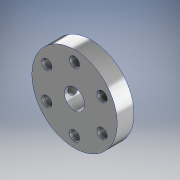
# Autodesk Inventor part: motor_axle_mounting_hub_6_mm
Saved by Autodesk Inventor 2016 (Build 200138000, 138)
## iProperties
Created: 2016-04-24
Part Number: motor_axle_mounting_hub_6_mm
Material: Aluminum 6061
Document SubType Name: Modeling
Designer: Henrik Samuelsson
Density: 2.7 g/cm^3
Appearance: Aluminum - Flat
Author: Henrik Samuelsson
Autodesk Inventor part; units mm, degrees
ref_plane "YZ Plane" through (0, 0, 0) normal (1, 0, 0) x (0, 1, 0)
ref_plane "XZ Plane" through (0, 0, 0) normal (0, 1, 0) x (-1, 0, 0)
ref_plane "XY Plane" through (0, 0, 0) normal (0, 0, 1) x (1, 0, 0)
sketch "Sketch1" plane through (0, 0, 0) normal (0, 1, 0) x (-1, 0, 0)
  circle A0 centre (0, 0) radius 12.7
  circle A1 centre (8.2272, -4.75) radius 1.5
  circle A2 centre (8.2272, 4.75) radius 1.5
  circle A3 centre (0, 9.5) radius 1.5
  circle A4 centre (-8.2272, 4.75) radius 1.5
  circle A5 centre (-8.2272, -4.75) radius 1.5
  circle A6 centre (0, -9.5) radius 1.5
  dimension "d0" = 25.4
  dimension "d1" = 3
  dimension "d3" = 9.5
  dimension "d6" = 360
  dimension "d20" = 0
  constraints: 7 centre point, 3 coincident, 17 other
  measures "d0" diameter of A0
  measures "d1" diameter of A1
  measures "d3" distance of A1.centre point (0, 0)
  measures "d20" horizontal distance of point (0, 0) A6.centre
extrude "Extrusion1" add sketch "Sketch1" along normal blind 5
sketch "Sketch2" plane through (0, 0, 0) normal (0, 1, 0) x (-1, 0, 0)
  circle A0 centre (0, 0) radius 3
  dimension "d10" = 6
  constraints: 1 centre point, 1 coincident
  measures "d10" diameter of A0
extrude "Extrusion2" cut sketch "Sketch2" along normal through all
sketch "Sketch3" plane through (0, 5, 0) normal (0, 1, 0) x (1, 0, 0)
  circle A0 centre (0, 0) radius 3
  circle A1 centre (0, 0) radius 6
  dimension "d13" = 12
  constraints: 2 centre point, 2 coincident
  measures "d13" diameter of A1
extrude "Extrusion3" add sketch "Sketch3" along normal blind 4.2
sketch "Sketch5" plane through (0, 0, 0) normal (1, 0, 0) x (0, 1, 0)
  circle A0 centre (2.5, 0) radius 1.5
  point P0 (0, 0)
  dimension "d21" = 3
  dimension "d22" = 2.5
  dimension "d23" = 0
  constraints: 1 centre point
  measures "d21" diameter of A0
  measures "d22" distance of point (0, 0) A0.centre
  measures "d23" vertical distance of point (0, 0) A0.centre
extrude "Extrusion4" cut sketch "Sketch5" against normal through all
sketch "Sketch6" plane through (0, 0, 0) normal (1, 0, 0) x (0, 1, 0)
  circle A0 centre (7.1, 0) radius 1.5
  point P0 (0, 0)
  dimension "d26" = 3
  dimension "d27" = 7.1
  dimension "d28" = 0
  constraints: 1 centre point
  measures "d26" diameter of A0
  measures "d27" distance of point (0, 0) A0.centre
  measures "d28" vertical distance of point (0, 0) A0.centre
extrude "Extrusion5" cut sketch "Sketch6" against normal through all
body "Solid1"
